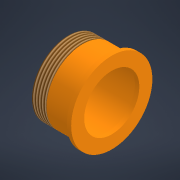
# Autodesk Inventor part: 030
Saved by Autodesk Inventor 2022 (Build 260153000, 153)
## iProperties
Created: 2022-04-04
Part Number: 030
Material: Aluminum 6061
Document SubType Name: Modeling
Designer: Vinicius Miguel
Density: 2.7 g/cm^3
Appearance: Orange
Mass: 5.38202 g
Surface Area: 28.7927 cm^2
Volume: 1.99334 cm^3
Author: Vinicius Miguel
Autodesk Inventor part; units mm, degrees
ref_plane "YZ Plane" through (0, 0, 0) normal (1, 0, 0) x (0, 1, 0)
ref_plane "XZ Plane" through (0, 0, 0) normal (0, 1, 0) x (-1, 0, 0)
ref_plane "XY Plane" through (0, 0, 0) normal (0, 0, 1) x (1, 0, 0)
sketch "Sketch1" plane through (0, 0, 0) normal (0, 1, 0) x (-1, 0, 0)
  line L0 (0, 0) -> (15, 0)
  line L1 (1.5, -11) -> (15, -11)
  line L2 (1.5, -11) -> (1.5, -9.5)
  line L3 (1.5, -9.5) -> (0, -9.5)
  line L4 (0, -9.5) -> (0, -14)
  line L5 (0, -14) -> (1.5, -14)
  line L6 (1.5, -14) -> (1.5, -12.5)
  line L7 (1.5, -12.5) -> (15, -12.5)
  line L8 (15, -12.5) -> (15, -11)
  dimension "d0" = 1.5
  dimension "d1" = 1.5
  dimension "d2" = 1.5
  dimension "d4" = 1.5
  dimension "d5" = 15
  dimension "d7" = 19
  dimension "d8" = 22
  constraints: 18 end point, 5 perpendicular, 2 horizontal, 2 point on line, 2 vertical alignment, 1 vertical
  measures "d0" distance of L1.start L2.end
  measures "d1" distance of L5.end L6.end
  measures "d2" distance of L4.end L5.end
  measures "d4" distance of L7.end L1.end
  measures "d5" distance of L0.start L0.end
  measures "d7" diameter of L3 L0
  measures "d8" diameter of L1 L0
revolve "Revolution1" add sketch "Sketch1" angle 360 about axis through (0, 0, 0) along (-1, 0, 0)
thread "Thread1" size "M25x1" class "6g" standard "ANSI Metric M Profile" length 5
body "Solid1"
